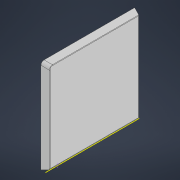
# Autodesk Inventor part: N__side_sticker
Saved by Autodesk Inventor 2022 (Build 260153070, 153G)
## iProperties
Created: 2021-11-16
Part Number: N__side_sticker
Material: Типовые
Document SubType Name: Modeling
Designer: kalugin_a
Density: 1 g/cm^3
Appearance: По умолчанию
Author: kalugin_a
Autodesk Inventor part; units mm, degrees
ref_plane "YZ Plane" through (0, 0, 0) normal (1, 0, 0) x (0, 1, 0)
ref_plane "XZ Plane" through (0, 0, 0) normal (0, 1, 0) x (-1, 0, 0)
ref_plane "XY Plane" through (0, 0, 0) normal (0, 0, 1) x (1, 0, 0)
ref_plane "РабПлоскость1" through (203.4395, -285.3633, -641.5751) normal (1, 0, 0) x (0, 1, 0)
sketch "Эскиз1" plane through (203.4395, -285.3633, -641.5751) normal (1, 0, 0) x (0, 1, 0)
  line L0 (-170.4999, 182.8495) -> (170.5001, 182.8495)
  line L1 (170.5001, 182.8495) -> (170.5001, -158.1505)
  line L2 (170.5001, -158.1505) -> (-170.4999, -158.1505)
  line L3 (-170.4999, -158.1505) -> (-170.4999, 182.8495)
  point P0 (285.3633, 641.5751)
  point P1 (49.5, 182.8495)
  point P2 (-170.4999, 137.85)
  dimension "d5" = 341
  dimension "d6" = 341
  constraints: 8 end point, 2 parallel, 2 point on line, 1 horizontal, 1 perpendicular
  measures "d5" distance of L0.end L1.end
  measures "d6" distance of L0.start L0.end
extrude "Выдавливание1" add sketch "Эскиз1" along normal blind 16
chamfer "Фаска1" distance 16 angle 45 1 edges at (219.4395, -114.8632, -629.2256)
sketch "Эскиз2" plane through (203.4395, -455.8632, -458.7256) normal (0, 0, 1) x (1, 0, 0)
  line L0 (16, 0) -> (16, 325) projected
  point P0 (-203.4395, 455.8632)
  point P1 (16, 220)
  constraints: 1 point on line
sketch "Эскиз3" plane through (219.4395, -285.3633, -641.5751) normal (1, 0, 0) x (0, 0, -1)
  line L0 (-182.8495, -170.4999) -> (158.1505, -170.4999) projected
  point P0 (-137.85, -170.4999)
  constraints: 1 point on line
chamfer "Фаска2" distance 16 angle 45 1 edges at (219.4395, -293.3631, -458.7256)
fillet "Сопряжение1" radius 16 2 edges at (203.4395, -114.8632, -458.7256) (211.4395, -122.8631, -466.7255)
fillet "Сопряжение2" radius 3 5 edges at (219.4395, -133.8946, -477.757) (219.4395, -299.02, -474.7255) (219.4395, -130.8631, -642.8824) (219.4395, -293.3631, -799.7256) (219.4395, -455.8632, -637.2255)
